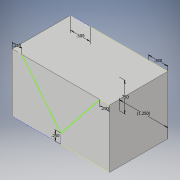
# Autodesk Inventor part: LoftCut
Saved by Autodesk Inventor 2017 (Build 210142000, 142)
## iProperties
Created: 2020-02-11
Part Number: LoftCut
Material: Generic
Document SubType Name: Modeling
Designer: 10042265
Density: 1 g/cm^3
Appearance: Default
Author: 10042265
Autodesk Inventor part; units mm, degrees
ref_plane "YZ Plane" through (0, 0, 0) normal (1, 0, 0) x (0, 1, 0)
ref_plane "XZ Plane" through (0, 0, 0) normal (0, 1, 0) x (-1, 0, 0)
ref_plane "XY Plane" through (0, 0, 0) normal (0, 0, 1) x (1, 0, 0)
sketch "Sketch1" plane through (0, 0, 0) normal (0, 0, 1) x (1, 0, 0)
  line L0 (0, 0) -> (63.5, 0)
  line L1 (63.5, 0) -> (63.5, 38.1)
  line L2 (63.5, 38.1) -> (0, 38.1)
  line L3 (0, 38.1) -> (0, 0)
  dimension "d0" = 63.5
  dimension "d1" = 38.1
  constraints: 8 end point, 3 perpendicular, 1 horizontal
  measures "d0" distance of L0.start L0.end
  measures "d1" distance of L0.end L1.end
extrude "Extrusion1" add sketch "Sketch1" along normal blind 38.1
sketch "Sketch3" plane through (0, 0, 38.1) normal (0, 0, 1) x (1, 0, 0)
  line L0 (0.001, 37.9851) -> (6.35, 38.1) construction
  line L1 (0, 0) -> (31.75, 0) construction
  line L2 (0, 0) -> (63.5, 0) construction
  line L3 (31.75, 0) -> (31.75, 6.35) construction
  line L4 (63.5, 38.1) -> (57.15, 38.1) construction
  line L5 (57.15, 38.1) -> (31.75, 6.35)
  line L6 (31.75, 6.35) -> (6.35, 38.1)
  dimension "d4" = 6.35
  dimension "d5" = 6.35
  dimension "d6" = 6.35
  constraints: 12 end point, 1 equal length, 1 midpoint, 1 perpendicular
  measures "d4" distance of L0.start L0.end
  measures "d5" distance of L1.end L3.end
  measures "d6" distance of L4.start L4.end
sketch "Sketch4" plane through (0, 0, 0) normal (0, 0, -1) x (-1, 0, 0)
  line L0 (-63.4999, 38.0548) -> (-50.8, 38.1) construction
  line L1 (-63.5, 38.1) -> (0, 38.1) construction
  line L2 (0, 38.1) -> (0, 0) construction
  line L3 (0, 38.1) -> (-12.7, 38.1) construction
  line L4 (0, 0) -> (-63.5, 0) construction
  line L5 (-63.5, 0) -> (-31.75, 0) construction
  line L6 (-31.75, 0) -> (-31.75, 19.05) construction
  line L7 (-31.75, 19.05) -> (-12.7, 38.1)
  line L8 (-31.75, 19.05) -> (-50.8, 38.1)
  dimension "d7" = 12.7
  dimension "d8" = 12.7
  dimension "d9" = 31.75
  dimension "d10" = 19.05
  constraints: 12 end point, 2 point on line, 1 midpoint, 1 perpendicular, 1 vertical
  measures "d7" distance of L0.start L0.end
  measures "d8" distance of L1.end L3.end
  measures "d9" distance of L4.end L5.end
  measures "d10" distance of L5.end L6.end
body "Solid1"
